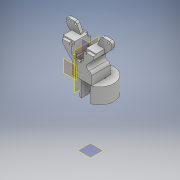
# Autodesk Inventor part: base_gripper_v3
Saved by Autodesk Inventor 2018 (Build 220112000, 112)
## iProperties
Created: 2018-02-12
Part Number: base_gripper_v3
Material: Generic
Document SubType Name: Modeling
Designer: Bardo91
Density: 1 g/cm^3
Appearance: Default
Author: Bardo91
Autodesk Inventor part; units mm, degrees
ref_plane "YZ Plane" through (0, 0, 0) normal (1, 0, 0) x (0, 1, 0)
ref_plane "XZ Plane" through (0, 0, 0) normal (0, 1, 0) x (-1, 0, 0)
ref_plane "XY Plane" through (0, 0, 0) normal (0, 0, 1) x (1, 0, 0)
sketch "Sketch1" plane through (0, 0, 0) normal (0, 0, 1) x (1, 0, 0)
  line L0 (0, 0) -> (18, 0)
  line L1 (18, 0) -> (18, 32)
  line L2 (18, 32) -> (0, 32)
  line L3 (0, 32) -> (0, 0)
  dimension "d0" = 18
  dimension "d1" = 32
  constraints: 8 end point, 2 perpendicular, 1 horizontal, 1 vertical
  measures "d0" distance of L0.start L0.end
  measures "d1" distance of L0.end L1.end
extrude "base" add sketch "Sketch1" along normal blind 25
sketch "Sketch2" plane through (0, 0, 25) normal (0, 0, 1) x (1, 0, 0)
  line L0 (18, 32) -> (0, 32) projected
  line L1 (9, 32) -> (9, 0)
  line L2 (9, 16) -> (9, 27.5)
  line L3 (9, 16) -> (20.5, 16) construction
  line L4 (9, 27.5) -> (15.25, 27.5)
  line L5 (15.25, 27.5) -> (15.25, 4.5)
  line L6 (15.25, 4.5) -> (2.75, 4.5)
  line L7 (2.75, 4.5) -> (2.75, 27.5)
  line L8 (2.75, 27.5) -> (9, 27.5)
  line L9 (0, 0) -> (18, 0) projected
  dimension "d4" = 11.5
  dimension "d5" = 90
  dimension "d6" = 6.25
  dimension "d7" = 23
  dimension "d8" = 12.5
  constraints: 16 end point, 6 perpendicular, 3 midpoint, 1 collinear, 1 horizontal, 1 point on line, 1 vertical
  measures "d4" distance of L2.start L2.end
  measures "d5" angle of L3 L2
  measures "d6" distance of L2.end L4.end
  measures "d7" distance of L4.end L5.end
  measures "d8" distance of L5.end L6.end
extrude "servo_place" cut sketch "Sketch2" against normal blind 18
ref_plane "Work Plane1" through (9, 22, -120) normal (0, 0, -1) x (-1, 0, 0)
sketch "Sketch6" plane through (0, 0, 25) normal (0, 0, 1) x (1, 0, 0)
  line L0 (0, 32) -> (0, 0)
  line L1 (2.75, 27.5) -> (15.25, 27.5)
  line L2 (0, 32) -> (2.75, 32)
  line L3 (2.75, 32) -> (2.75, 27.5)
  line L4 (2.75, 27.5) -> (0, 27.5)
  line L5 (0, 27.5) -> (0, 32)
  line L6 (18, 32) -> (15.256294, 32)
  line L7 (15.256294, 32) -> (15.256294, 27.5)
  line L8 (15.256294, 27.5) -> (18, 27.5)
  line L9 (18, 27.5) -> (18, 32)
  line L10 (15.25, 27.5) -> (15.25, 4.5)
  line L11 (18, 0) -> (15.25, 0)
  line L12 (15.25, 0) -> (15.25, 4.5)
  line L13 (15.25, 4.5) -> (18, 4.5)
  line L14 (18, 4.5) -> (18, 0)
  line L15 (0, 0) -> (2.75, 0)
  line L16 (2.75, 0) -> (2.75, 4.5)
  line L17 (2.75, 4.5) -> (0, 4.5)
  line L18 (0, 4.5) -> (0, 0)
  constraints: 32 end point, 8 parallel, 4 horizontal, 4 perpendicular, 4 point on line
extrude "pilars_top" add sketch "Sketch6" along normal blind 15
sketch "Sketch9" plane through (0, 0, 40) normal (0, 0, 1) x (1, 0, 0)
  line L0 (0, 32) -> (0, 0) projected
  line L1 (18, 0) -> (18, 32) projected
  line L2 (0, 32) -> (18, 32)
  line L3 (18, 32) -> (18, 0)
  line L4 (18, 0) -> (0, 0)
  line L5 (0, 0) -> (0, 32)
  line L6 (18, 32) -> (36, 32)
  line L7 (36, 32) -> (36, 0)
  line L8 (36, 0) -> (18, 0)
  line L9 (0, 32) -> (-18, 32)
  line L10 (-18, 32) -> (-18, 0)
  line L11 (-18, 0) -> (0, 0)
  point P0 (0, 22)
  point P1 (18, 22)
  dimension "d39" = 18
  dimension "d40" = 18
  constraints: 20 end point, 5 perpendicular, 3 parallel, 1 horizontal, 1 point on line, 1 vertical
  measures "d39" distance of L1.end L6.end
  measures "d40" distance of L0.start L9.end
extrude "base_top" add sketch "Sketch9" along normal blind 5
sketch "Sketch10" plane through (0, 0, 45) normal (0, 0, 1) x (1, 0, 0)
  line L0 (18, 32) -> (0, 32)
  line L1 (15.293033, 32) -> (15.293033, 0)
  line L2 (15.25, 27.5) -> (15.25, 4.5)
  line L3 (15.256294, 27.5) -> (15.256294, 32)
  line L4 (15.256294, 32) -> (2.756294, 32)
  line L5 (36, 32) -> (-18, 32)
  line L6 (2.756294, 32) -> (2.756294, 0)
  line L7 (0, 0) -> (18, 0)
  line L8 (15.293033, 0) -> (2.756294, 0)
  dimension "d100" = 12.5
  constraints: 8 end point, 3 point on line, 1 collinear, 1 parallel, 1 perpendicular
  measures "d100" distance of L3.end L4.end
extrude "screw_hole" cut sketch "Sketch10" against normal blind 5
ref_plane "Work Plane2" through (0, 0, 10) normal (0, 0, -1) x (-1, 0, 0)
ref_plane "Work Plane6" through (0, -4, 10) normal (0, -1, 0) x (1, 0, 0)
ref_plane "Work Plane5" through (0, 36, 10) normal (0, 1, 0) x (1, 0, 0)
sketch "Sketch16" plane through (2.75, 0, 25) normal (0, -1, 0) x (1, 0, 0)
  line L0 (12.506294, 20) -> (15.25, 20)
  line L1 (15.25, 20) -> (33.25, 20)
  line L2 (15.25, 20) -> (15.25, -5)
  line L3 (15.25, -25) -> (15.25, 15)
  line L4 (15.25, -5) -> (33.25, 15)
  point P0 (-2.75, -25)
  point P1 (15.25, -7)
  dimension "d95" = 25
  constraints: 6 end point, 1 horizontal, 1 midpoint
  measures "d95" distance of L0.end L2.end
sketch "Sketch16 outline for Extrusion16" plane through (2.75, 0, 25) normal (0, -1, 0) x (1, 0, 0)
  line L0 (33.25, 15) -> (15.25, 20)
  line L1 (15.25, -5) -> (33.25, 15)
  line L2 (15.25, 20) -> (15.25, -5)
extrude "Extrusion16" add sketch "Sketch16 outline for Extrusion16" against normal blind 4.6
ref_plane "Work Plane3" through (2.75, 16, 25) normal (0, 1, 0) x (1, 0, 0)
ref_plane "Work Plane4" through (9, -4, -17) normal (1, 0, 0) x (0, 0, -1)
mirror "Mirror1" about plane through (2.75, 16, 25) normal (0, 1, 0) of "Extrusion16"
mirror "Mirror2" about plane through (9, -4, -17) normal (1, 0, 0) of "Extrusion16", "Mirror1"
sketch "Sketch18" plane through (2.75, 0, 25) normal (0, -1, 0) x (1, 0, 0)
  line L0 (12.5, 0) -> (0, 0)
  line L1 (6.25, 0) -> (6.25, 5)
  line L2 (6.25, 5) -> (-3.75, 5)
  line L3 (-3.75, 5) -> (-3.75, 20)
  line L4 (-20.75, 20) -> (0.006294, 20)
  line L5 (-3.75, 20) -> (16.25, 20)
  line L6 (16.25, 20) -> (16.25, 5)
  line L7 (16.25, 5) -> (6.25, 5)
  point P0 (-2.75, -25)
  dimension "d105" = 5
  dimension "d106" = 10
  dimension "d107" = 20
  constraints: 12 end point, 5 perpendicular, 2 point on line, 1 midpoint, 1 vertical
  measures "d105" distance of L1.start L1.end
  measures "d106" distance of L1.end L2.end
  measures "d107" distance of L3.end L5.end
extrude "Extrusion18" cut sketch "Sketch18" against normal through all
sketch "Sketch19" plane through (0, 0, 45) normal (0, 0, 1) x (1, 0, 0)
  line L0 (-1, 0) -> (-1, 32) projected
  line L1 (-1, 32) -> (-6, 32)
  line L2 (0, 32) -> (-18, 32) projected
  line L3 (-6, 32) -> (-6, 0)
  line L4 (-6, 0) -> (24, 0)
  line L5 (24, 0) -> (24, 32)
  line L6 (24, 32) -> (-1, 32)
  point P0 (0, 0)
  dimension "d110" = 5
  dimension "d111" = 30
  constraints: 10 end point, 4 perpendicular, 2 point on line
  measures "d110" distance of L0.end L1.end
  measures "d111" distance of L3.end L4.end
extrude "Extrusion19" cut sketch "Sketch19" against normal blind 3
sketch "Sketch20" plane through (0, 0, 42) normal (0, 0, 1) x (1, 0, 0)
  line L0 (-6, 32) -> (-1, 32) projected
  line L1 (-6, 32) -> (-3.5, 32)
  line L2 (-3.5, 32) -> (-3.5, 29.5)
  circle A0 centre (-3.5, 29.5) radius 1.4
  point P0 (0, 0)
  dimension "d114" = 2.5
  dimension "d115" = 2.5
  dimension "d116" = 2.8
  constraints: 4 end point, 1 centre point, 1 coincident, 1 midpoint, 1 perpendicular
  measures "d114" distance of L0.start L1.end
  measures "d115" distance of L1.end L2.end
  measures "d116" diameter of A0
extrude "Extrusion20" cut sketch "Sketch20" against normal blind 5
mirror "Mirror3" about plane through (9, -4, -17) normal (1, 0, 0) of "Extrusion20"
mirror "Mirror4" about plane through (2.75, 16, 25) normal (0, 1, 0) of "Extrusion20", "Mirror3"
sketch "Sketch21" plane through (0, 0, 25) normal (0, 0, 1) x (1, 0, 0)
  line L0 (2.75, 4.5) -> (2.75, 27.5) projected
  line L1 (2.75, 16) -> (2.75, 27.75)
  line L2 (2.75, 27.75) -> (15.25, 27.75)
  line L3 (15.25, 27.75) -> (15.25, 4.25)
  line L4 (15.25, 27.5) -> (15.25, 4.5) projected
  line L5 (15.25, 4.25) -> (2.75, 4.25)
  line L6 (2.75, 4.25) -> (2.75, 16)
  point P0 (0, 0)
  dimension "d119" = 11.75
  dimension "d120" = 12.5
  dimension "d121" = 23.5
  dimension "d122" = 12.5
  constraints: 10 end point, 2 collinear, 1 midpoint, 1 perpendicular, 1 point on line
  measures "d119" distance of L1.start L1.end
  measures "d120" distance of L1.end L2.end
  measures "d121" distance of L2.end L3.end
  measures "d122" distance of L3.end L5.end
extrude "Extrusion21" cut sketch "Sketch21" against normal up to surface (18 mm away)
sketch "Sketch22" plane through (2.75, 27.75, 25) normal (0, -1, 0) x (1, 0, 0)
  line L0 (12.5, 0) -> (12.5, -18) projected
  line L1 (0, -18) -> (12.5, -18) projected
  line L2 (12.5, -18) -> (0, -18)
  line L3 (0, -18) -> (0, -11)
  line L4 (0, -11) -> (12.5, -11)
  line L5 (12.5, -11) -> (12.5, -18)
  point P0 (-2.75, -25)
  dimension "d125" = 7
  constraints: 8 end point, 3 perpendicular, 1 collinear
  measures "d125" distance of L1.start L3.end
extrude "Extrusion22" cut sketch "Sketch22" against normal through all
sketch "Sketch23" plane through (18, 27.4, 20) normal (0, -1, 0) x (1, 0, 0)
  line L0 (18, 20) -> (1, 20)
  line L1 (18, 20) -> (1, 20)
  line L2 (0, 0) -> (18, 20)
  line L3 (18, 20) -> (0, 0)
  line L4 (0, 0) -> (0, 5)
  line L5 (0, 0) -> (0, 27)
  line L6 (0, 27) -> (18, 27)
  line L7 (18, 27) -> (18, 20)
  line L8 (-38.593165, 22.881294) -> (-18, 0)
  line L9 (-18, 0) -> (-36, 20)
  line L10 (-18, 0) -> (-18, 27)
  line L11 (-18, 27) -> (-38.593165, 27)
  line L12 (-38.593165, 27) -> (-38.593165, 22.881294)
  point P0 (-18, -20)
  dimension "d131" = 27
  dimension "d132" = 27
  constraints: 18 end point, 4 perpendicular, 3 collinear, 2 point on line, 1 horizontal, 1 vertical
  measures "d131" distance of L5.start L5.end
  measures "d132" distance of L8.end L10.end
extrude "Extrusion23" add sketch "Sketch23" along normal up to surface (22.8 mm away)
sketch "Sketch11" plane through (0, 0, 45) normal (0, 0, 1) x (1, 0, 0)
  circle A0 centre (9, 22) radius 6
  line L0 (9, 22) -> (36, 22)
  line L1 (36, 0) -> (36, 32)
  line L2 (36, 22) -> (36, 24.5)
  line L3 (36, 24.5) -> (31, 24.5)
  line L4 (31, 24.5) -> (31, 19.5)
  line L5 (31, 19.5) -> (36, 19.5)
  line L6 (36, 19.5) -> (36, 24.5)
  line L7 (9, 22) -> (9, 34.070881)
  line L8 (-18, 22) -> (-18, 24.5)
  line L9 (-18, 24.5) -> (-13, 24.5)
  line L10 (-13, 24.5) -> (-13, 19.5)
  line L11 (-13, 19.5) -> (-18, 19.5)
  line L12 (-18, 19.5) -> (-18, 24.5)
  dimension "d60" = 2.5
  dimension "d61" = 5
  dimension "d62" = 5
  constraints: 24 end point, 5 symmetric about line, 3 perpendicular, 3 point on line, 1 collinear, 1 horizontal, 1 vertical
  measures "d60" distance of L0.end L2.end
  measures "d61" distance of L2.end L3.end
  measures "d62" distance of L3.end L4.end
extrude "Extrusion11" cut sketch "Sketch11" against normal through all contours L4 L3 L1 L0 | L0 L1 L5 L4 | L8 L9 L10 L11 L12
sketch "Sketch24" plane through (31, 19.5, 45) normal (0, 1, 0) x (1, 0, 0)
  line L0 (0, 0) -> (10, 0)
  line L1 (0, 0) -> (5, 0)
  circle A0 centre (2, -14) radius 1.75
  line L2 (2, -14) -> (12, -14)
  circle A1 centre (12, -14) radius 1.75
  line L3 (-7, 0) -> (5, 0)
  line L4 (-7, 0) -> (-7, -3)
  line L5 (-7, -3) -> (-0.660726, -16.594617)
  line L6 (-0.660726, -16.594617) -> (-0.660726, -17.594617)
  line L7 (-0.660726, -17.594617) -> (17.339274, -17.594617)
  line L8 (17.339274, -17.594617) -> (17.339274, -9.594617)
  line L9 (17.339274, -9.594617) -> (14.803564, -4.15677)
  line L10 (5, 5) -> (5, 0)
  line L11 (0, 3.24715) -> (0, 0)
  line L12 (5, 5) -> (0, 10.555556)
  line L13 (14.803564, -4.15677) -> (0, 10.555556)
  line L14 (0, 10.555556) -> (0, 3.24715)
  line L15 (-22, 90.32132) -> (-22, -37.927922)
  line L16 (5, -2) -> (-13, -2)
  point P0 (-31, 45)
  dimension "d135" = 10
  dimension "d137" = 3.5
  dimension "d138" = 10
  dimension "d139" = 3.5
  dimension "d140" = 3
  dimension "d141" = 15
  dimension "d142" = 155
  dimension "d143" = 1
  dimension "d144" = 18
  dimension "d145" = 8
  dimension "d146" = 6
  dimension "d229" = 24
  dimension "d230" = 12
  constraints: 22 end point, 2 centre point, 2 collinear, 2 parallel, 2 perpendicular, 1 coincident, 1 horizontal, 1 vertical
  measures "d135" distance of L0.start L0.end
  measures "d137" diameter of A0
  measures "d138" distance of L2.start L2.end
  measures "d139" diameter of A1
  measures "d140" distance of L3.start L4.end
  measures "d141" distance of L4.end L5.end
  measures "d142" angle of L5 L4
  measures "d143" distance of L5.end L6.end
  measures "d144" distance of L6.end L7.end
  measures "d145" distance of L7.end L8.end
  measures "d146" distance of L8.end L9.end
  measures "d229" distance from line of L15 L2.start
  measures "d230" distance from line of L16 L2.start
extrude "Extrusion24" add sketch "Sketch24" along normal blind 5
fillet "Fillet5" radius 4 6 edges at (48.3393, 22, 62.5946) (30.3393, 22, 62.5946) (30.3393, 22, 61.5946) (48.3393, 22, 54.5946) (45.8036, 22, 49.1568) (24, 22, 48)
mirror "Mirror5" about plane through (9, -4, -17) normal (1, 0, 0) of "Extrusion24", "Fillet5"
sketch "Sketch25" plane through (0, 0, 25) normal (0, 0, 1) x (1, 0, 0)
  line L0 (2.75, 4.5) -> (2.75, 27.5) projected
  line L1 (2.75, 16) -> (2.75, 4.5)
  line L2 (2.75, 4.5) -> (15.25, 4.5)
  line L3 (15.25, 4.25) -> (2.75, 4.25) projected
  line L4 (15.25, 4.5) -> (15.25, 27.5)
  line L5 (15.25, 27.75) -> (15.25, 4.5) projected
  line L6 (15.25, 27.5) -> (2.75, 27.5)
  line L7 (2.75, 27.5) -> (2.75, 16)
  point P0 (0, 0)
  dimension "d150" = 11.5
  dimension "d151" = 23
  constraints: 10 end point, 3 collinear, 1 midpoint, 1 parallel, 1 perpendicular, 1 point on line
  measures "d150" distance of L1.start L1.end
  measures "d151" distance of L2.end L4.end
extrude "Extrusion25" cut sketch "Sketch25" against normal up to surface (18 mm away)
sketch "Sketch26" plane through (18, 0, 0) normal (1, 0, 0) x (0, 0, -1)
  line L0 (0, 0) -> (-20, 0) projected
  line L1 (0, 0) -> (-20, 0)
  line L2 (-20, 0) -> (-20, 32) projected
  line L3 (-20, 0) -> (-20, 32)
  line L4 (0, 32) -> (-20, 32) projected
  line L5 (-20, 32) -> (0, 32)
  line L6 (0, 32) -> (0, 0)
  constraints: 8 end point, 2 perpendicular, 1 collinear, 1 horizontal
extrude "Extrusion26" add sketch "Sketch26" along normal blind 15
sketch "Sketch27" plane through (0, 0, 0) normal (0, 0, -1) x (-1, 0, 0)
  line L0 (-33, 0) -> (-33, 32) projected
  line L1 (-33, 16) -> (-30, 16)
  line L2 (-30, 16) -> (-30, 28.5)
  line L3 (-30, 28.5) -> (-17.5, 28.5)
  line L4 (-17.5, 28.5) -> (-17.5, 3.5)
  line L5 (-18, 32) -> (-18, 0) projected
  line L6 (-17.5, 3.5) -> (-30, 3.5)
  line L7 (-30, 3.5) -> (-30, 16)
  point P0 (0, 0)
  dimension "d156" = 3
  dimension "d157" = 12.5
  dimension "d158" = 12.5
  dimension "d159" = 90
  dimension "d160" = 25
  dimension "d161" = 90
  dimension "d162" = 12.5
  constraints: 12 end point, 2 perpendicular, 1 horizontal, 1 midpoint, 1 parallel, 1 point on line
  measures "d156" distance of L1.start L1.end
  measures "d157" distance of L1.end L2.end
  measures "d158" distance of L2.end L3.end
  measures "d159" angle of L2 L3
  measures "d160" distance of L3.end L4.end
  measures "d161" angle of L3 L4
  measures "d162" distance of L4.end L6.end
extrude "Extrusion27" cut sketch "Sketch27" against normal blind 18
fillet "Fillet6" radius 5 2 edges at (18, 16, 20) (33, 16, 20)
sketch "Sketch28" plane through (0, 0, 0) normal (0, 0, -1) x (-1, 0, 0)
  line L0 (-30, 28.5) -> (-17.5, 28.5)
  line L1 (-23.75, 28.5) -> (-23.75, 30.3)
  line L2 (-25.510341, 32) -> (-25.510341, 0)
  line L3 (-23.75, 28.5) -> (-21.95, 28.5) construction
  circle A0 centre (-23.75, 30.3) radius 1
  line L4 (-17.5, 3.5) -> (-30, 3.5)
  line L5 (-23.75, 3.5) -> (-23.75, 1.7)
  line L6 (-23.75, 3.5) -> (-21.95, 3.5) construction
  circle A1 centre (-23.75, 1.7) radius 1
  point P0 (0, 0)
  dimension "d166" = 1.8
  dimension "d167" = 90
  dimension "d168" = 2
  dimension "d169" = 1.8
  dimension "d170" = 90
  dimension "d171" = 2
  constraints: 8 end point, 2 centre point, 2 coincident, 2 horizontal, 2 midpoint, 2 perpendicular, 1 parallel, 1 vertical
  measures "d166" distance of L1.start L1.end
  measures "d167" angle of L3 L1
  measures "d168" diameter of A0
  measures "d169" distance of L5.start L5.end
  measures "d170" angle of L5 L6
  measures "d171" diameter of A1
extrude "Extrusion28" cut sketch "Sketch28" against normal up to surface (20 mm away)
sketch "Sketch29" plane through (17.5, 28.5, 0) normal (0, -1, 0) x (1, 0, 0)
  line L0 (0, 18) -> (12.5, 18) projected
  line L1 (0, 18) -> (0, 11)
  line L2 (0, 0) -> (0, 18) projected
  line L3 (0, 11) -> (12.5, 11)
  line L4 (12.5, 0) -> (12.5, 18) projected
  line L5 (12.5, 11) -> (12.5, 18)
  line L6 (12.5, 18) -> (0, 18)
  point P0 (-17.5, 0)
  dimension "d174" = 7
  constraints: 8 end point, 2 perpendicular, 2 point on line, 1 collinear
  measures "d174" distance of L0.start L1.end
extrude "Extrusion29" cut sketch "Sketch29" against normal blind 18
sketch "Sketch30" plane through (0, 0, 0) normal (0, 0, -1) x (-1, 0, 0)
  circle A0 centre (-23.75, 30.3) radius 1
  line L0 (-23.75, 30.3) -> (-23.75, 22.8)
  line L1 (-24, 32) -> (-24, 0)
  line L2 (-23.75, 30.3) -> (-16.25, 30.3) construction
  circle A1 centre (-23.75, 22.8) radius 25
  circle A2 centre (-23.75, 22.8) radius 27.5
  line L3 (-36, 32) -> (-24, 32)
  line L4 (-31, 32) -> (-29, 32) construction
  line L5 (-31.151614, 34.382684) -> (-16.151614, 34.382684)
  line L6 (-16.151614, 34.382684) -> (-16.151614, -1.017316)
  line L7 (-16.151614, 34.382684) -> (19.248386, 34.382684) construction
  line L8 (-16.151614, -1.017316) -> (-31.348386, -1.017316)
  line L9 (-31.348386, -1.017316) -> (-31.348386, 31.951098)
  line L10 (-31.348386, 31.951098) -> (-31.348386, 34.382684)
  line L11 (-31.151614, 34.382684) -> (-31.348386, 34.382684)
  point P0 (0, 0)
  dimension "d177" = 7.5
  dimension "d178" = 90
  dimension "d179" = 50
  dimension "d180" = 55
  dimension "d187" = 90
  dimension "d221" = 35.4
  dimension "d222" = 15
  dimension "d223" = 32.96841
  constraints: 20 end point, 5 perpendicular, 4 horizontal, 2 centre point, 2 coincident, 2 point on circle, 1 parallel, 1 point on line, 1 vertical
  measures "d177" distance of L0.start L0.end
  measures "d178" angle of L0 L2
  measures "d179" diameter of A1
  measures "d180" diameter of A2
  measures "d187" angle of L6 L7
  measures "d221" distance of L5.end L6.end
  measures "d222" distance of L5.start L5.end
  measures "d223" distance of L8.end L9.end
sketch "Sketch32" plane through (0, 0, 0) normal (0, 0, -1) x (-1, 0, 0)
  circle A0 centre (-23.75, 30.3) radius 1
  line L0 (-23.75, 30.3) -> (-23.75, 22.8)
  line L1 (-25.510341, 32) -> (-25.510341, 0)
  line L2 (-23.75, 30.3) -> (-16.25, 30.3) construction
  circle A1 centre (-23.75, 22.8) radius 9.7
  circle A2 centre (-23.75, 22.8) radius 25
  point P0 (0, 0)
  dimension "d190" = 7.5
  dimension "d191" = 90
  dimension "d192" = 19.4
  dimension "d193" = 50
  constraints: 4 end point, 2 centre point, 2 coincident, 1 horizontal, 1 parallel, 1 perpendicular
  measures "d190" distance of L0.start L0.end
  measures "d191" angle of L0 L2
  measures "d192" diameter of A1
  measures "d193" diameter of A2
extrude "Extrusion32" add sketch "Sketch32" along normal blind 18 contours A2
sketch "Sketch33" plane through (23.75, 22.8, -18) normal (0, 0, -1) x (-1, 0, 0)
  circle A0 centre (0, 0) radius 12.2
  circle A1 centre (0, 0) radius 25
  point P0 (23.75, -22.8)
  dimension "d196" = 24.4
  dimension "d197" = 50
  constraints: 2 centre point, 1 coincident
  measures "d196" diameter of A0
  measures "d197" diameter of A1
extrude "Extrusion33" add sketch "Sketch33" along normal blind 9
sketch "Sketch34" plane through (0, 0, 25) normal (0, 0, 1) x (1, 0, 0)
  line L0 (2.75, 4.25) -> (15.25, 4.25) projected
  line L1 (9, 4.25) -> (9, 1.75)
  line L2 (9, 1.75) -> (12.5, 1.75)
  line L3 (9, 1.75) -> (12.5, 1.75) construction
  line L4 (12.5, 1.75) -> (5.5, 1.75)
  circle A0 centre (12.5, 1.75) radius 1
  circle A1 centre (5.5, 1.75) radius 1
  line L5 (2.75, 27.75) -> (15.25, 27.75) projected
  line L6 (9, 27.75) -> (9, 30.25)
  line L7 (9, 30.25) -> (5.5, 30.25)
  line L8 (5.5, 30.25) -> (12.5, 30.25)
  circle A2 centre (12.5, 30.25) radius 1
  circle A3 centre (5.5, 30.25) radius 1
  point P0 (0, 0)
  dimension "d200" = 2.5
  dimension "d201" = 3.5
  dimension "d202" = 0
  dimension "d203" = 7
  dimension "d204" = 2
  dimension "d205" = 2
  dimension "d208" = 2.5
  dimension "d209" = 3.5
  dimension "d210" = 7
  dimension "d211" = 2
  dimension "d212" = 2
  constraints: 14 end point, 4 centre point, 4 coincident, 2 horizontal, 2 midpoint, 2 point on line, 2 vertical, 1 collinear, 1 perpendicular
  measures "d200" distance of L1.start L1.end
  measures "d201" distance of L1.end L2.end
  measures "d202" distance between parallel lines of L2 L3
  measures "d203" distance of L2.end L4.end
  measures "d204" diameter of A0
  measures "d205" diameter of A1
  measures "d208" distance of L6.start L6.end
  measures "d209" distance of L6.end L7.end
  measures "d210" distance of L7.end L8.end
  measures "d211" diameter of A2
  measures "d212" diameter of A3
extrude "Extrusion34" cut sketch "Sketch34" against normal blind 9
sketch "Sketch35" plane through (-20.593165, 27.4, 47) normal (0, 0, 1) x (1, 0, 0)
  line L0 (38.593165, -22.8) -> (39.593165, -22.8)
  line L1 (19.593165, -27.4) -> (19.593165, -22.8)
  line L2 (39.593165, -22.8) -> (19.593165, -22.8)
  line L3 (19.593165, 0) -> (19.593165, 4.6)
  line L4 (19.593165, -22.8) -> (19.593165, 0)
  line L5 (14.593165, 0) -> (19.593165, 0)
  line L6 (39.593165, 0) -> (38.593165, 0)
  line L7 (19.593165, 0) -> (39.593165, 0)
  line L8 (39.593165, 0) -> (39.593165, -22.8)
  point P0 (20.593165, -27.4)
  constraints: 8 end point, 3 perpendicular, 1 collinear
extrude "Extrusion35" cut sketch "Sketch35" against normal up to surface (22 mm away)
sketch "Sketch36" plane through (0, 0, 0) normal (0, 0, -1) x (-1, 0, 0)
  line L0 (-30, 28.5) -> (-30, 32)
  line L1 (-30, 3.5) -> (-30, 15.381948)
  line L2 (-30, 28.5) -> (-30, 3.5)
  line L3 (-17.5, 3.5) -> (-30, 3.5)
  line L4 (-30, 3.5) -> (-17.5, 3.5)
  line L5 (-17.5, 3.5) -> (-17.5, 28.5)
  line L6 (-17.5, 32) -> (-17.5, 3.5)
  line L7 (-30, 28.5) -> (-17.5, 28.5)
  line L8 (-19, 27.4) -> (-19, 32)
  line L9 (-30, 3.5) -> (-30, 0)
  line L10 (-30, 0) -> (-17.5, 0)
  line L11 (-19, 0) -> (-15.25, 0)
  line L12 (-17.5, 3.5) -> (-17.5, 0)
  line L13 (-30, 28.5) -> (-30, 32)
  line L14 (-30, 32) -> (-17.5, 32)
  line L15 (-30, 32) -> (-17.5, 32)
  line L16 (-17.5, 32) -> (-17.5, 28.5)
  point P0 (0, 0)
  constraints: 20 end point, 4 collinear, 2 perpendicular, 2 point on line, 1 horizontal, 1 vertical
extrude "Extrusion36" cut sketch "Sketch36" along normal through all
sketch "Sketch37" plane through (0, 0, -18) normal (0, 0, -1) x (-1, 0, 0)
  arc A0 (-17.5, 12.322524) -> (-30, 12.322524) centre (-23.75, 22.8) ccw
  circle A1 centre (-23.75, 22.8) radius 12.2
  circle A2 centre (-23.75, 22.8) radius 11
  point P0 (0, 0)
  dimension "d217" = 22
  dimension "d228" = 24.4
  constraints: 2 centre point, 2 coincident
  measures "d217" diameter of A2
  measures "d228" diameter of A1
extrude "Extrusion37" add sketch "Sketch37" along normal blind 4
sketch "Sketch38" plane through (0, 0, 0) normal (0, 0, -1) x (-1, 0, 0)
  line L0 (-17.5, 28.5) -> (-17.5, 32)
  line L1 (-28.613406, 0) -> (-33, 0)
  line L2 (-17.5, 32) -> (-30.069471, 32)
  line L3 (-30.069471, 32) -> (-30.069471, 0)
  line L4 (-30.069471, 0) -> (-17.5, 0)
  line L5 (-17.5, 0) -> (-17.5, 32)
  line L6 (-15.5, 34) -> (-32.069471, 34)
  line L7 (-32.069471, 34) -> (-32.069471, -2)
  line L8 (-32.069471, -2) -> (-15.5, -2)
  line L9 (-15.5, -2) -> (-15.5, 34)
  line L10 (-15.5, -2) -> (-15.5, -3)
  line L11 (-15.5, -3) -> (-32.069471, -3)
  line L12 (-32.069471, -3) -> (-32.069471, -2)
  point P0 (0, 0)
  dimension "d224" = 2
  dimension "d227" = 1
  constraints: 22 end point, 4 parallel, 4 perpendicular, 1 horizontal, 1 point on line, 1 vertical, 3 other
  measures "d224" distance between parallel lines of L5 L9
  measures "d227" distance of L8.end L10.end
extrude "Extrusion38" cut sketch "Sketch38" along normal through all contours L5 L4 L1 L3 L2 L0 | L9 L8 L7 L6 | L10 L11 L12 L8
equation "\"d151\" = 2 * d150"
body "Solid1"
